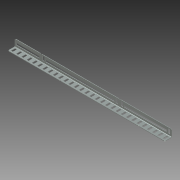
# Autodesk Inventor part: Slotted Angle 30 Hole
Saved by Autodesk Inventor 2013 (Build 170138000, 138)
## iProperties
Category: Structure
Company: Autodesk Inc.
Created: 2012-04-12
Part Number: Slotted Angle 30 Hole
Document SubType Name: Sheet Metal
Designer: Autodesk Inc.
Density: 7.85 g/cm^3
Sheet Metal Rule: Default
Material: Steel
Catalog Web Link: http://www.vexrobotics.com/segmented-angle.html
Vendor: VEX
Mass: 97.4246 g
Surface Area: 227.297 cm^2
Volume: 12.4108 cm^3
Author: Autodesk Inc.
Autodesk Inventor part; units mm, degrees
ref_plane "YZ Plane" through (0, 0, 0) normal (1, 0, 0) x (0, 1, 0)
ref_plane "XZ Plane" through (0, 0, 0) normal (0, 1, 0) x (-1, 0, 0)
ref_plane "XY Plane" through (0, 0, 0) normal (0, 0, 1) x (1, 0, 0)
sketch "Sketch1" plane through (0, 0, 0) normal (0, 0, 1) x (1, 0, 0)
  line L0 (-27.0361, 17.9126) -> (-22.4641, 17.9126)
  line L1 (-22.4641, 17.9126) -> (-22.4641, 8.1336)
  line L2 (-22.4641, 8.1336) -> (-27.0361, 8.1336)
  line L3 (-27.0361, 8.1336) -> (-27.0361, 17.9126)
  line L4 (-31.1001, 19.4366) -> (-31.1001, 4.8316)
  line L5 (349.8999, 19.4366) -> (349.8999, 4.8316)
  line L6 (-29.1951, 21.3416) -> (30.4949, 21.3416)
  line L7 (-31.1001, 4.8316) -> (349.8999, 4.8316)
  line L8 (32.3999, 19.4366) -> (32.3999, 4.8316)
  line L9 (32.3999, 19.4366) -> (30.4949, 21.3416)
  line L10 (-29.1951, 21.3416) -> (-31.1001, 19.4366)
  line L11 (-14.3361, 17.9126) -> (-9.7641, 17.9126)
  line L12 (-9.7641, 17.9126) -> (-9.7641, 8.1336)
  line L13 (-9.7641, 8.1336) -> (-14.3361, 8.1336)
  line L14 (-14.3361, 8.1336) -> (-14.3361, 17.9126)
  line L15 (-1.6361, 17.9126) -> (2.9359, 17.9126)
  line L16 (2.9359, 17.9126) -> (2.9359, 8.1336)
  line L17 (2.9359, 8.1336) -> (-1.6361, 8.1336)
  line L18 (-1.6361, 8.1336) -> (-1.6361, 17.9126)
  line L19 (11.0639, 17.9126) -> (15.6359, 17.9126)
  line L20 (15.6359, 17.9126) -> (15.6359, 8.1336)
  line L21 (15.6359, 8.1336) -> (11.0639, 8.1336)
  line L22 (11.0639, 8.1336) -> (11.0639, 17.9126)
  line L23 (23.7639, 17.9126) -> (28.3359, 17.9126)
  line L24 (28.3359, 17.9126) -> (28.3359, 8.1336)
  line L25 (28.3359, 8.1336) -> (23.7639, 8.1336)
  line L26 (23.7639, 8.1336) -> (23.7639, 17.9126)
  line L27 (36.4639, 17.9126) -> (41.0359, 17.9126)
  line L28 (41.0359, 17.9126) -> (41.0359, 8.1336)
  line L29 (41.0359, 8.1336) -> (36.4639, 8.1336)
  line L30 (36.4639, 8.1336) -> (36.4639, 17.9126)
  line L31 (49.1639, 17.9126) -> (53.7359, 17.9126)
  line L32 (53.7359, 17.9126) -> (53.7359, 8.1336)
  line L33 (53.7359, 8.1336) -> (49.1639, 8.1336)
  line L34 (49.1639, 8.1336) -> (49.1639, 17.9126)
  line L35 (61.8639, 17.9126) -> (66.4359, 17.9126)
  line L36 (66.4359, 17.9126) -> (66.4359, 8.1336)
  line L37 (66.4359, 8.1336) -> (61.8639, 8.1336)
  line L38 (61.8639, 8.1336) -> (61.8639, 17.9126)
  line L39 (74.5639, 17.9126) -> (79.1359, 17.9126)
  line L40 (79.1359, 17.9126) -> (79.1359, 8.1336)
  line L41 (79.1359, 8.1336) -> (74.5639, 8.1336)
  line L42 (74.5639, 8.1336) -> (74.5639, 17.9126)
  line L43 (87.2639, 17.9126) -> (91.8359, 17.9126)
  line L44 (91.8359, 17.9126) -> (91.8359, 8.1336)
  line L45 (91.8359, 8.1336) -> (87.2639, 8.1336)
  line L46 (87.2639, 8.1336) -> (87.2639, 17.9126)
  line L47 (99.9639, 17.9126) -> (104.5359, 17.9126)
  line L48 (104.5359, 17.9126) -> (104.5359, 8.1336)
  line L49 (104.5359, 8.1336) -> (99.9639, 8.1336)
  line L50 (99.9639, 8.1336) -> (99.9639, 17.9126)
  line L51 (112.6639, 17.9126) -> (117.2359, 17.9126)
  line L52 (117.2359, 17.9126) -> (117.2359, 8.1336)
  line L53 (117.2359, 8.1336) -> (112.6639, 8.1336)
  line L54 (112.6639, 8.1336) -> (112.6639, 17.9126)
  line L55 (125.3639, 17.9126) -> (129.9359, 17.9126)
  line L56 (129.9359, 17.9126) -> (129.9359, 8.1336)
  line L57 (129.9359, 8.1336) -> (125.3639, 8.1336)
  line L58 (125.3639, 8.1336) -> (125.3639, 17.9126)
  line L59 (138.0639, 17.9126) -> (142.6359, 17.9126)
  line L60 (142.6359, 17.9126) -> (142.6359, 8.1336)
  line L61 (142.6359, 8.1336) -> (138.0639, 8.1336)
  line L62 (138.0639, 8.1336) -> (138.0639, 17.9126)
  line L63 (150.7639, 17.9126) -> (155.3359, 17.9126)
  line L64 (155.3359, 17.9126) -> (155.3359, 8.1336)
  line L65 (155.3359, 8.1336) -> (150.7639, 8.1336)
  line L66 (150.7639, 8.1336) -> (150.7639, 17.9126)
  line L67 (163.4639, 17.9126) -> (168.0359, 17.9126)
  line L68 (168.0359, 17.9126) -> (168.0359, 8.1336)
  line L69 (168.0359, 8.1336) -> (163.4639, 8.1336)
  line L70 (163.4639, 8.1336) -> (163.4639, 17.9126)
  line L71 (176.1639, 17.9126) -> (180.7359, 17.9126)
  line L72 (180.7359, 17.9126) -> (180.7359, 8.1336)
  line L73 (180.7359, 8.1336) -> (176.1639, 8.1336)
  line L74 (176.1639, 8.1336) -> (176.1639, 17.9126)
  line L75 (188.8639, 17.9126) -> (193.4359, 17.9126)
  line L76 (193.4359, 17.9126) -> (193.4359, 8.1336)
  line L77 (193.4359, 8.1336) -> (188.8639, 8.1336)
  line L78 (188.8639, 8.1336) -> (188.8639, 17.9126)
  line L79 (201.5639, 17.9126) -> (206.1359, 17.9126)
  line L80 (206.1359, 17.9126) -> (206.1359, 8.1336)
  line L81 (206.1359, 8.1336) -> (201.5639, 8.1336)
  line L82 (201.5639, 8.1336) -> (201.5639, 17.9126)
  line L83 (214.2639, 17.9126) -> (218.8359, 17.9126)
  line L84 (218.8359, 17.9126) -> (218.8359, 8.1336)
  line L85 (218.8359, 8.1336) -> (214.2639, 8.1336)
  line L86 (214.2639, 8.1336) -> (214.2639, 17.9126)
  line L87 (226.9639, 17.9126) -> (231.5359, 17.9126)
  line L88 (231.5359, 17.9126) -> (231.5359, 8.1336)
  line L89 (231.5359, 8.1336) -> (226.9639, 8.1336)
  line L90 (226.9639, 8.1336) -> (226.9639, 17.9126)
  line L91 (239.6639, 17.9126) -> (244.2359, 17.9126)
  line L92 (244.2359, 17.9126) -> (244.2359, 8.1336)
  line L93 (244.2359, 8.1336) -> (239.6639, 8.1336)
  line L94 (239.6639, 8.1336) -> (239.6639, 17.9126)
  line L95 (252.3639, 17.9126) -> (256.9359, 17.9126)
  line L96 (256.9359, 17.9126) -> (256.9359, 8.1336)
  line L97 (256.9359, 8.1336) -> (252.3639, 8.1336)
  line L98 (252.3639, 8.1336) -> (252.3639, 17.9126)
  line L99 (265.0639, 17.9126) -> (269.6359, 17.9126)
  line L100 (269.6359, 17.9126) -> (269.6359, 8.1336)
  line L101 (269.6359, 8.1336) -> (265.0639, 8.1336)
  line L102 (265.0639, 8.1336) -> (265.0639, 17.9126)
  line L103 (277.7639, 17.9126) -> (282.3359, 17.9126)
  line L104 (282.3359, 17.9126) -> (282.3359, 8.1336)
  line L105 (282.3359, 8.1336) -> (277.7639, 8.1336)
  line L106 (277.7639, 8.1336) -> (277.7639, 17.9126)
  line L107 (290.4639, 17.9126) -> (295.0359, 17.9126)
  line L108 (295.0359, 17.9126) -> (295.0359, 8.1336)
  line L109 (295.0359, 8.1336) -> (290.4639, 8.1336)
  line L110 (290.4639, 8.1336) -> (290.4639, 17.9126)
  line L111 (303.1639, 17.9126) -> (307.7359, 17.9126)
  line L112 (307.7359, 17.9126) -> (307.7359, 8.1336)
  line L113 (307.7359, 8.1336) -> (303.1639, 8.1336)
  line L114 (303.1639, 8.1336) -> (303.1639, 17.9126)
  line L115 (315.8639, 17.9126) -> (320.4359, 17.9126)
  line L116 (320.4359, 17.9126) -> (320.4359, 8.1336)
  line L117 (320.4359, 8.1336) -> (315.8639, 8.1336)
  line L118 (315.8639, 8.1336) -> (315.8639, 17.9126)
  line L119 (328.5639, 17.9126) -> (333.1359, 17.9126)
  line L120 (333.1359, 17.9126) -> (333.1359, 8.1336)
  line L121 (333.1359, 8.1336) -> (328.5639, 8.1336)
  line L122 (328.5639, 8.1336) -> (328.5639, 17.9126)
  line L123 (341.2639, 17.9126) -> (345.8359, 17.9126)
  line L124 (345.8359, 17.9126) -> (345.8359, 8.1336)
  line L125 (345.8359, 8.1336) -> (341.2639, 8.1336)
  line L126 (341.2639, 8.1336) -> (341.2639, 17.9126)
  line L127 (32.3999, 19.4366) -> (34.3049, 21.3416)
  line L128 (34.3049, 21.3416) -> (220.9949, 21.3416)
  line L129 (222.8999, 19.4366) -> (222.8999, 4.8316)
  line L130 (222.8999, 19.4366) -> (220.9949, 21.3416)
  line L131 (222.8999, 19.4366) -> (224.8049, 21.3416)
  line L132 (224.8049, 21.3416) -> (347.9949, 21.3416)
  line L133 (349.8999, 19.4366) -> (347.9949, 21.3416)
  point P0 (-31.1001, 21.3416)
  point P1 (349.8999, 21.3416)
  point P2 (32.3999, 21.3416)
  point P3 (222.8999, 21.3416)
  dimension "d1" = 4.064
  dimension "d2" = 9.779
  dimension "d3" = 4.572
  dimension "d12" = 16.51
  dimension "d14" = 1.905
  dimension "d15" = 1.905
  dimension "d16" = 1.905
  dimension "d17" = 1.905
  dimension "d20" = 12.7
  dimension "d25" = 4.064
  dimension "d26" = 1.905
  dimension "d27" = 1.905
  dimension "d28" = 1.905
  dimension "d29" = 1.905
  measures "d1" distance between parallel lines of L3 L4
  measures "d2" distance between parallel lines of L2 L0
  measures "d3" distance of L0.start L0.end
  measures "d12" distance of point (-31.1, 21.342) L4.end
  measures "d14" distance of L8.start point (32.4, 21.342)
  measures "d15" distance of L6.end point (32.4, 21.342)
  measures "d16" distance of L6.start point (-31.1, 21.342)
  measures "d17" distance of L4.start point (-31.1, 21.342)
  measures "d20" distance of L2.end L14.start
  measures "d25" distance between parallel lines of L129 L84
  measures "d26" distance of L129.start point (222.9, 21.342)
  measures "d27" distance of L128.end point (222.9, 21.342)
  measures "d28" distance of L5.start point (349.9, 21.342)
  measures "d29" distance of L132.end point (349.9, 21.342)
extrude "Plate1" add sketch "Sketch1" along normal blind 1.27
sketch "Sketch2" plane through (349.8999, 4.8316, 1.27) normal (0, 1, 0) x (-1, 0, 0)
  line L0 (0, 0) -> (381, 0)
  line L1 (381, 0) -> (381, 16.51)
  line L2 (381, 16.51) -> (0, 16.51)
  line L3 (0, 16.51) -> (0, 0)
  constraints: 6 end point, 1 horizontal, 1 perpendicular, 1 vertical
sheet face with bend "Flange1" sketch "Sketch2" thickness 1.27 toward (0, -1, 0) bend radius 0.8636 relief straight relief width 1.27 relief depth 0.635
bend "Bend1"
chamfer "Corner Chamfer1" distance 1.905 angle 45 2 edges at (-31.1001, 4.1966, 17.78) (349.8999, 4.1966, 17.78)
sketch "Sketch3" plane through (-31.1001, 4.8316, 2.1336) normal (0, 1, 0) x (1, 0, 0)
  line L0 (381, -13.7414) -> (381, 0) projected
  line L1 (0, 0) -> (0, -13.7414) projected
  line L2 (1.905, -15.6464) -> (379.095, -15.6464) projected
  line L3 (3.302, -7.0104) -> (60.198, -7.0104)
  line L4 (60.198, -7.0104) -> (60.198, -11.5824)
  line L5 (60.198, -11.5824) -> (3.302, -11.5824)
  line L6 (3.302, -11.5824) -> (3.302, -7.0104)
  line L7 (1.905, -15.6464) -> (63.5, -15.6464)
  line L8 (63.5, -13.7414) -> (63.5, -1.0855)
  line L9 (61.595, -15.6464) -> (51.3359, -15.6464)
  line L10 (63.5, -13.7414) -> (61.595, -15.6464)
  line L11 (63.5, -13.7414) -> (65.405, -15.6464)
  line L12 (67.564, -2.4384) -> (72.136, -2.4384)
  line L13 (72.136, -2.4384) -> (72.136, -12.2174)
  line L14 (72.136, -12.2174) -> (67.564, -12.2174)
  line L15 (67.564, -12.2174) -> (67.564, -2.4384)
  line L16 (75.184, -7.0104) -> (242.316, -7.0104)
  line L17 (242.316, -7.0104) -> (242.316, -11.5824)
  line L18 (242.316, -11.5824) -> (75.184, -11.5824)
  line L19 (75.184, -11.5824) -> (75.184, -7.0104)
  line L20 (245.364, -2.4384) -> (249.936, -2.4384)
  line L21 (249.936, -2.4384) -> (249.936, -12.2174)
  line L22 (249.936, -12.2174) -> (245.364, -12.2174)
  line L23 (245.364, -12.2174) -> (245.364, -2.4384)
  line L24 (254, 0.235) -> (254, -13.7414)
  line L25 (238.0435, -15.6464) -> (252.095, -15.6464)
  line L26 (252.095, -15.6464) -> (254, -13.7414)
  line L27 (255.905, -15.6464) -> (254, -13.7414)
  line L28 (258.064, -2.4384) -> (262.636, -2.4384)
  line L29 (262.636, -2.4384) -> (262.636, -12.2174)
  line L30 (262.636, -12.2174) -> (258.064, -12.2174)
  line L31 (258.064, -12.2174) -> (258.064, -2.4384)
  line L32 (265.684, -7.0104) -> (369.316, -7.0104)
  line L33 (369.316, -7.0104) -> (369.316, -11.5824)
  line L34 (369.316, -11.5824) -> (265.684, -11.5824)
  line L35 (265.684, -11.5824) -> (265.684, -7.0104)
  line L36 (372.364, -2.4384) -> (376.936, -2.4384)
  line L37 (376.936, -2.4384) -> (376.936, -12.2174)
  line L38 (376.936, -12.2174) -> (372.364, -12.2174)
  line L39 (372.364, -12.2174) -> (372.364, -2.4384)
  line L40 (0, 0) -> (381, 0) projected
  line L41 (61.595, -15.6464) -> (65.405, -15.6464)
  line L42 (252.095, -15.6464) -> (255.905, -15.6464)
  point P0 (63.5, -15.6464)
  point P1 (254, -15.6464)
  dimension "d41" = 3.302
  dimension "d42" = 4.064
  dimension "d43" = 4.572
  dimension "d45" = 1.905
  dimension "d46" = 1.905
  dimension "d47" = 0
  dimension "d48" = 4.064
  dimension "d49" = 4.572
  dimension "d50" = 3.429
  dimension "d51" = 9.779
  dimension "d52" = 3.048
  dimension "d53" = 4.572
  dimension "d54" = 177.8
  dimension "d55" = 3.048
  dimension "d56" = 4.572
  dimension "d58" = 1.905
  dimension "d59" = 1.905
  dimension "d60" = 0
  dimension "d61" = 4.064
  dimension "d62" = 4.064
  dimension "d63" = 4.572
  dimension "d64" = 3.048
  dimension "d65" = 4.064
  dimension "d67" = 3.048
  dimension "d68" = 4.572
  dimension "d81" = 3.302
  constraints: 78 end point, 16 parallel, 11 collinear, 10 perpendicular, 7 horizontal, 6 point on line, 2 symmetric about line
  measures "d41" distance between parallel lines of L1 L6
  measures "d42" distance between parallel lines of L2 L5
  measures "d43" distance between parallel lines of L3 L5
  measures "d45" distance of L8.start point (63.5, -15.646)
  measures "d46" distance of L9.start point (63.5, -15.646)
  measures "d47" distance between parallel lines of L7 L9
  measures "d48" distance between parallel lines of L15 L8
  measures "d49" distance of L12.start L12.end
  measures "d50" distance between parallel lines of L2 L14
  measures "d51" distance of L12.end L13.end
  measures "d52" distance between parallel lines of L19 L13
  measures "d53" distance between parallel lines of L13 L15
  measures "d54" distance between parallel lines of L15 L23
  measures "d55" distance between parallel lines of L23 L17
  measures "d56" distance of L21.end L22.end
  measures "d58" distance of L25.end point (254, -15.646)
  measures "d59" distance of L24.end point (254, -15.646)
  measures "d60" distance between parallel lines of L2 L25
  measures "d61" distance between parallel lines of L24 L21
  measures "d62" distance between parallel lines of L31 L24
  measures "d63" distance between parallel lines of L31 L29
  measures "d64" distance between parallel lines of L35 L29
  measures "d65" distance between parallel lines of L0 L37
  measures "d67" distance between parallel lines of L33 L39
  measures "d68" distance between parallel lines of L37 L39
  measures "d81" distance between parallel lines of L8 L4
cut "Cut1" [suppressed]
sketch "Sketch4" plane through (-31.1001, 4.8316, 2.1336) normal (0, 1, 0) x (1, 0, 0)
  line L0 (62.992, 3.2766) -> (64.008, 3.2766)
  line L1 (64.008, 3.2766) -> (64.008, -0.5334)
  line L2 (64.008, -0.5334) -> (62.992, -0.5334)
  line L3 (62.992, -0.5334) -> (62.992, 3.2766)
  line L4 (253.492, 3.2766) -> (254.508, 3.2766)
  line L5 (254.508, 3.2766) -> (254.508, -0.5334)
  line L6 (254.508, -0.5334) -> (253.492, -0.5334)
  line L7 (253.492, -0.5334) -> (253.492, 3.2766)
  point P0 (63.5, -13.7414)
  point P1 (254, -13.7414)
  dimension "d71" = 0.508
  dimension "d72" = 0.508
  dimension "d73" = 13.208
  dimension "d74" = 3.81
  dimension "d77" = 0.508
  dimension "d78" = 0.508
  dimension "d79" = 3.81
  dimension "d80" = 13.208
  constraints: 16 end point, 4 parallel, 2 horizontal, 2 perpendicular
  measures "d71" distance from line of L1 point (63.5, -13.741)
  measures "d72" distance from line of point (63.5, -13.741) L3
  measures "d73" distance from line of point (63.5, -13.741) L2
  measures "d74" distance between parallel lines of L0 L2
  measures "d77" distance from line of L5 point (254, -13.741)
  measures "d78" distance from line of L7 point (254, -13.741)
  measures "d79" distance between parallel lines of L4 L6
  measures "d80" distance from line of point (254, -13.741) L6
extrude "Extrusion1" [suppressed]
sketch "Sketch5" plane through (34.3049, 21.3416, 1.27) normal (0, 0, 1) x (1, 0, 0)
  line L0 (306.959, -13.208) -> (306.959, -3.429) projected
  line L1 (306.959, -3.429) -> (311.531, -3.429) projected
  line L2 (311.531, -3.429) -> (311.531, -13.208) projected
  circle A0 centre (309.245, -5.715) radius 2.286
  point P0 (-34.3049, -21.3416)
  constraints: 3 tangent, 1 centre point
surface extrude "ExtrusionSrf1" sketch "Sketch5" against normal up to surface (1.27 mm away) shown no curves A0
sketch "Sketch6" plane through (34.3049, 21.3416, 1.27) normal (0, 0, 1) x (1, 0, 0)
  line L0 (306.959, -13.208) -> (306.959, -3.429) projected
  line L1 (311.531, -3.429) -> (311.531, -13.208) projected
  line L2 (311.531, -13.208) -> (306.959, -13.208) projected
  circle A0 centre (309.245, -10.922) radius 2.286
  point P0 (-34.3049, -21.3416)
  constraints: 3 tangent, 1 centre point
surface extrude "ExtrusionSrf2" sketch "Sketch6" against normal up to surface (1.27 mm away) shown no curves A0
pattern_linear "Rectangular Pattern1" count 30 spacing 12.7 along (-1, 0, 0) of "ExtrusionSrf1", "ExtrusionSrf2"
sketch "Sketch7" plane through (349.8999, 3.5616, 2.1336) normal (0, -1, 0) x (1, 0, 0)
  line L0 (-0.913, 17.1604) -> (-0.913, 5.1828)
  line L1 (-381.3206, 3.419) -> (-381.3206, 17.1604)
  line L2 (-2.4974, 1.7638) -> (-379.6874, 1.7638)
  line L3 (-3.302, 8.636) -> (-60.198, 8.636)
  line L4 (-60.198, 8.636) -> (-60.198, 4.064)
  line L5 (-60.198, 4.064) -> (-3.302, 4.064)
  line L6 (-3.302, 4.064) -> (-3.302, 8.636)
  line L7 (-2.4974, 1.7638) -> (-64.0924, 1.7638)
  line L8 (-64.0924, 3.6688) -> (-64.0924, 16.3247)
  line L9 (-62.1874, 1.7638) -> (-51.9283, 1.7638)
  line L10 (-64.0924, 3.6688) -> (-62.1874, 1.7638)
  line L11 (-64.0924, 3.6688) -> (-65.9974, 1.7638)
  line L12 (-67.564, 13.208) -> (-72.136, 13.208)
  line L13 (-72.136, 13.208) -> (-72.136, 3.429)
  line L14 (-72.136, 3.429) -> (-67.564, 3.429)
  line L15 (-67.564, 3.429) -> (-67.564, 13.208)
  line L16 (-75.184, 8.636) -> (-242.316, 8.636)
  line L17 (-242.316, 8.636) -> (-242.316, 4.064)
  line L18 (-242.316, 4.064) -> (-75.184, 4.064)
  line L19 (-75.184, 4.064) -> (-75.184, 8.636)
  line L20 (-245.364, 13.208) -> (-249.936, 13.208)
  line L21 (-249.936, 13.208) -> (-249.936, 3.429)
  line L22 (-249.936, 3.429) -> (-245.364, 3.429)
  line L23 (-245.364, 3.429) -> (-245.364, 13.208)
  line L24 (-254.3206, 17.3954) -> (-254.3206, 3.419)
  line L25 (-238.3641, 1.514) -> (-252.4156, 1.514)
  line L26 (-252.4156, 1.514) -> (-254.3206, 3.419)
  line L27 (-256.2256, 1.514) -> (-254.3206, 3.419)
  line L28 (-258.064, 13.208) -> (-262.636, 13.208)
  line L29 (-262.636, 13.208) -> (-262.636, 3.429)
  line L30 (-262.636, 3.429) -> (-258.064, 3.429)
  line L31 (-258.064, 3.429) -> (-258.064, 13.208)
  line L32 (-265.684, 8.636) -> (-369.316, 8.636)
  line L33 (-369.316, 8.636) -> (-369.316, 4.064)
  line L34 (-369.316, 4.064) -> (-265.684, 4.064)
  line L35 (-265.684, 4.064) -> (-265.684, 8.636)
  line L36 (-372.364, 13.208) -> (-376.936, 13.208)
  line L37 (-376.936, 13.208) -> (-376.936, 3.429)
  line L38 (-376.936, 3.429) -> (-372.364, 3.429)
  line L39 (-372.364, 3.429) -> (-372.364, 13.208)
  line L40 (-0.913, 17.1604) -> (-381.3206, 17.1604)
  line L41 (-62.1874, 1.7638) -> (-65.9974, 1.7638)
  line L42 (-252.4156, 1.514) -> (-256.2256, 1.514)
  line L43 (-381, 13.7414) -> (-381, 15.6464)
  line L44 (-379.095, 15.6464) -> (-381, 15.6464)
  line L45 (-379.095, 15.6464) -> (-1.905, 15.6464) projected
  line L46 (-125.095, 15.6464) -> (-127, 13.7414) projected
  line L47 (-128.905, 15.6464) -> (-127, 13.7414) projected
  line L48 (-256.2256, 15.6464) -> (-254.3206, 13.7414)
  line L49 (-254.3206, 13.7414) -> (-252.4156, 15.6464)
  line L50 (-65.9974, 15.6464) -> (-64.0924, 13.7414)
  line L51 (-64.0924, 13.7414) -> (-62.1874, 15.6464)
  point P0 (-349.8999, -2.1336)
  point P1 (-64.0924, 1.7638)
  point P2 (-254.3206, 1.514)
  dimension "d231" = 127
  dimension "d232" = 1.905
  dimension "d233" = 1.905
  dimension "d234" = 63.1794
  dimension "d235" = 1.905
  dimension "d236" = 1.905
  constraints: 98 end point, 12 point on line, 4 perpendicular
  measures "d231" distance between parallel lines of L24 L1
  measures "d232" horizontal distance of L48.start L48.end
  measures "d233" distance from line of L48.end L45
  measures "d234" distance between parallel lines of L8 L0
  measures "d235" horizontal distance of L50.start L50.end
  measures "d236" horizontal distance of L50.start L50.end
extrude "Cut2" cut sketch "Sketch7" against normal blind 1.27 contours L50 L45 L8 | L8 L45 L51 | L48 L45 L24 | L24 L45 L49 | L6 L5 L4 L3 | L15 L14 L13 L12 | L19 L18 L17 L16 | L23 L22 L21 L20 | L31 L30 L29 L28 | L35 L34 L33 L32 | L39 L38 L37 L36
sketch "Sketch8" plane through (-31.1001, 4.8316, 2.1336) normal (0, 1, 0) x (1, 0, 0)
  line L0 (138.684, -4.064) -> (305.816, -4.064) projected
  line L1 (305.816, -4.064) -> (305.816, -8.636) projected
  line L2 (305.816, -8.636) -> (138.684, -8.636) projected
  line L3 (138.684, -8.636) -> (138.684, -4.064) projected
  line L4 (11.684, -8.636) -> (11.684, -4.064) projected
  line L5 (11.684, -4.064) -> (115.316, -4.064) projected
  line L6 (115.316, -4.064) -> (115.316, -8.636) projected
  line L7 (115.316, -8.636) -> (11.684, -8.636) projected
  line L8 (320.802, -8.636) -> (320.802, -4.064) projected
  line L9 (320.802, -4.064) -> (377.698, -4.064) projected
  line L10 (377.698, -4.064) -> (377.698, -8.636) projected
  line L11 (377.698, -8.636) -> (320.802, -8.636) projected
  line L12 (8.636, -3.429) -> (8.636, -13.208) projected
  line L13 (8.636, -13.208) -> (4.064, -13.208) projected
  line L14 (4.064, -13.208) -> (4.064, -3.429) projected
  line L15 (4.064, -3.429) -> (8.636, -3.429) projected
  line L16 (131.064, -13.208) -> (131.064, -3.429) projected
  line L17 (131.064, -3.429) -> (135.636, -3.429) projected
  line L18 (135.636, -3.429) -> (135.636, -13.208) projected
  line L19 (135.636, -13.208) -> (131.064, -13.208) projected
  line L20 (118.364, -13.208) -> (118.364, -3.429) projected
  line L21 (118.364, -3.429) -> (122.936, -3.429) projected
  line L22 (122.936, -3.429) -> (122.936, -13.208) projected
  line L23 (122.936, -13.208) -> (118.364, -13.208) projected
  line L24 (308.864, -3.429) -> (313.436, -3.429) projected
  line L25 (313.436, -3.429) -> (313.436, -13.208) projected
  line L26 (313.436, -13.208) -> (308.864, -13.208) projected
  line L27 (308.864, -13.208) -> (308.864, -3.429) projected
  circle A0 centre (375.412, -6.35) radius 2.286
  circle A1 centre (323.088, -6.35) radius 2.286
  circle A2 centre (311.15, -10.922) radius 2.286
  circle A3 centre (311.15, -5.715) radius 2.286
  circle A4 centre (303.53, -6.35) radius 2.286
  circle A5 centre (140.97, -6.35) radius 2.286
  circle A6 centre (133.35, -10.922) radius 2.286
  circle A7 centre (133.35, -5.715) radius 2.286
  circle A8 centre (120.65, -10.922) radius 2.286
  circle A9 centre (120.65, -5.715) radius 2.286
  circle A10 centre (113.03, -6.35) radius 2.286
  circle A11 centre (13.97, -6.35) radius 2.286
  circle A12 centre (6.35, -10.922) radius 2.286
  circle A13 centre (6.35, -5.715) radius 2.286
  point P0 (31.1001, 2.1336)
  constraints: 42 tangent, 14 centre point
surface extrude "ExtrusionSrf61" sketch "Sketch8" against normal up to surface (1.27 mm away) shown no curves A0
surface extrude "ExtrusionSrf62" sketch "Sketch8" against normal up to surface (1.27 mm away) shown no curves A1
surface extrude "ExtrusionSrf63" sketch "Sketch8" against normal up to surface (1.27 mm away) shown no curves A2
surface extrude "ExtrusionSrf64" sketch "Sketch8" against normal up to surface (1.27 mm away) shown no curves A3
surface extrude "ExtrusionSrf65" sketch "Sketch8" against normal up to surface (1.27 mm away) shown no curves A4
surface extrude "ExtrusionSrf66" sketch "Sketch8" against normal up to surface (1.27 mm away) shown no curves A5
surface extrude "ExtrusionSrf67" sketch "Sketch8" against normal up to surface (1.27 mm away) shown no curves A6
surface extrude "ExtrusionSrf68" sketch "Sketch8" against normal up to surface (1.27 mm away) shown no curves A7
surface extrude "ExtrusionSrf69" sketch "Sketch8" against normal up to surface (1.27 mm away) shown no curves A8
surface extrude "ExtrusionSrf70" sketch "Sketch8" against normal up to surface (1.27 mm away) shown no curves A9
surface extrude "ExtrusionSrf71" sketch "Sketch8" against normal up to surface (1.27 mm away) shown no curves A10
surface extrude "ExtrusionSrf72" sketch "Sketch8" against normal up to surface (1.27 mm away) shown no curves A11
surface extrude "ExtrusionSrf73" sketch "Sketch8" against normal up to surface (1.27 mm away) shown no curves A12
surface extrude "ExtrusionSrf74" sketch "Sketch8" against normal up to surface (1.27 mm away) shown no curves A13
equation "\"d46\" = d45"
equation "\"d59\" = d58"
equation "\"d15\" = d14"
equation "\"d17\" = d16"
equation "\"d27\" = d26"
equation "\"d29\" = d28"
equation "\"d69\" = Thickness"
equation "\"d233\" = d232"
equation "\"d236\" = d235"
equation "\"d229\" = Thickness"
equation "\"d31\" = BendReliefWidth"
equation "\"d33\" = MinimumRemnant"
equation "\"d32\" = BendReliefDepth"
equation "\"d34\" = BendRadius"
equation "\"BendRadius\" = Thickness"
equation "\"BendReliefWidth\" = Thickness"
equation "\"BendReliefDepth\" = 0.5 * Thickness"
equation "\"CornerReliefSize\" = 4 * Thickness"
equation "\"MinimumRemnant\" = 2 * Thickness"
equation "\"TransitionRadius\" = BendRadius"
equation "\"d30\" = BendRadius"
equation "\"JacobiRadiusSize\" = Thickness"
equation "\"GapSize\" = Thickness"
equation "\"Thickness\" = 1.27"
body "Solid1"
body "Srf1"
body "Srf2"
body "Srf4"
body "Srf6"
body "Srf8"
body "Srf10"
body "Srf12"
body "Srf14"
body "Srf16"
body "Srf18"
body "Srf20"
body "Srf22"
body "Srf24"
body "Srf26"
body "Srf28"
body "Srf30"
body "Srf32"
body "Srf34"
body "Srf36"
body "Srf38"
body "Srf40"
body "Srf42"
body "Srf44"
body "Srf46"
body "Srf48"
body "Srf50"
body "Srf52"
body "Srf54"
body "Srf56"
body "Srf58"
body "Srf60"
body "Srf3"
body "Srf5"
body "Srf7"
body "Srf9"
body "Srf11"
body "Srf13"
body "Srf15"
body "Srf17"
body "Srf19"
body "Srf21"
body "Srf23"
body "Srf25"
body "Srf27"
body "Srf29"
body "Srf31"
body "Srf33"
body "Srf35"
body "Srf37"
body "Srf39"
body "Srf41"
body "Srf43"
body "Srf45"
body "Srf47"
body "Srf49"
body "Srf51"
body "Srf53"
body "Srf55"
body "Srf57"
body "Srf59"
body "Srf61"
body "Srf62"
body "Srf63"
body "Srf64"
body "Srf65"
body "Srf66"
body "Srf67"
body "Srf68"
body "Srf69"
body "Srf70"
body "Srf71"
body "Srf72"
body "Srf73"
body "Srf74"
